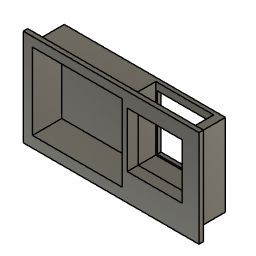
Insert v1 (Autodesk Fusion 360 design; units mm, degrees)
Autodesk Fusion 360 part; units mm, degrees
sketch "Sketch1" plane through (0, 0, 0) normal (0, 1, 0) x (1, 0, 0) in component "Component"
  line L0 (0, 0) -> (240, 0)
  line L1 (240, 0) -> (240, -132)
  line L2 (240, -132) -> (0, -132)
  line L3 (0, -132) -> (0, 0)
  dimension "d1" = 240
  dimension "d2" = 132
  constraint horizontal L0
  constraint vertical L1
  constraint horizontal L2
  constraint vertical L3
  constraint coincident L0.start L3.end
  measures "d1" distance of L0.start L0.end
  measures "d2" distance of L0.start L2.end
extrude "Extrude1" add sketch "Sketch1" along normal blind 6 in component "Component"
sketch "Sketch2" plane through (0, 6, 0) normal (0, 1, 0) x (-1, 0, 0) in component "Component"
  line L0 (0, 132) -> (-240, 132)
  line L1 (-240, 132) -> (-240, 0)
  line L2 (-240, 0) -> (0, 0)
  line L3 (0, 0) -> (0, 132)
  line L4 (-10, 10) -> (-230, 10)
  line L5 (-230, 10) -> (-230, 122)
  line L6 (-230, 122) -> (-10, 122)
  line L7 (-10, 122) -> (-10, 10)
  dimension "d5" = 220
  dimension "d6" = 112
  constraint horizontal L4
  constraint vertical L5
  constraint horizontal L6
  constraint vertical L7
  measures "d5" distance of L4.start L4.end
  measures "d6" distance of L4.start L6.end
extrude "Extrude2" add sketch "Sketch2" along normal blind 40 contours L4 L5 L6 L7 in component "Component"
sketch "Sketch3" plane through (0, 0, 0) normal (0, 1, 0) x (1, 0, 0) in component "Component"
  line L0 (12.5, -119.5) -> (225, -119.5)
  line L1 (225, -119.5) -> (225, -15)
  line L2 (225, -15) -> (12.5, -15)
  line L3 (12.5, -15) -> (12.5, -119.5)
  constraint horizontal L0
  constraint vertical L1
  constraint horizontal L2
  constraint vertical L3
extrude "Extrude3" cut sketch "Sketch3" along normal blind 40 in component "Component"
sketch "Sketch4" plane through (0, 0, 0) normal (0, 1, 0) x (1, 0, 0) in component "Component"
  line L0 (225, -15) -> (185, -15)
  line L1 (185, -15) -> (185, -120)
  line L2 (185, -120) -> (225, -120)
  line L3 (225, -120) -> (225, -15)
  constraint horizontal L0
  constraint vertical L1
  constraint horizontal L2
  constraint vertical L3
extrude "Extrude4" add 1 faces at (225, 13.3333, 84.6667) along direction (-1, 0, 0) blind 90 in component "Component"
sketch "Sketch5" plane through (0, 0, 0) normal (0, 1, 0) x (1, 0, 0) in component "Component"
  line L0 (140, -115) -> (219, -115)
  line L1 (219, -115) -> (219, -35)
  line L2 (219, -35) -> (140, -35)
  line L3 (140, -35) -> (140, -115)
  line L4 (140, -115) -> (220, -115)
  line L5 (220, -115) -> (220, -35)
  line L6 (220, -35) -> (140, -35)
  line L7 (140, -35) -> (140, -115)
  dimension "d13" = 80
  dimension "d14" = 80
  constraint horizontal L0
  constraint vertical L1
  constraint horizontal L2
  constraint vertical L3
  constraint horizontal L4
  constraint vertical L5
  constraint horizontal L6
  constraint vertical L7
  measures "d13" distance of L0.start L4.end
  measures "d14" distance of L0.start L2.end
extrude "Extrude5" cut sketch "Sketch5" along normal blind 50 contours L0 L1 L2 L3 L4 L6 L7 in component "Component"
sketch "Sketch6" plane through (219, 0, 0) normal (-1, 0, 0) x (0, -1, 0) in component "Component"
  line L0 (-46, 115) -> (-46, 35)
  line L1 (-46, 35) -> (0, 35)
  line L2 (0, 35) -> (0, 115)
  line L3 (0, 115) -> (-46, 115)
  line L4 (-46, 35) -> (-41, 35)
  line L5 (-41, 35) -> (-41, 37)
  line L6 (-41, 37) -> (-46, 37)
  line L7 (-46, 37) -> (-46, 35)
  constraint horizontal L4
  constraint vertical L5
  constraint horizontal L6
  constraint vertical L7
  constraint coincident L0.end L1.start
extrude "Extrude6" add sketch "Sketch6" along normal up to surface (79 mm away) contours L0 L1 L4 L5 L6 L7 in component "Component"
sketch "Sketch7" plane through (219, 0, 0) normal (-1, 0, 0) x (0, -1, 0) in component "Component"
  line L0 (-46, 37) -> (-41, 37)
  line L1 (-41, 37) -> (-41, 35)
  line L2 (-41, 35) -> (0, 35)
  line L3 (0, 35) -> (0, 115)
  line L4 (0, 115) -> (-46, 115)
  line L5 (-46, 115) -> (-46, 37)
  line L6 (-41, 37) -> (-15, 37)
  line L7 (-15, 37) -> (-15, 35)
  line L8 (-15, 35) -> (-41, 35)
  line L9 (-41, 35) -> (-41, 37)
  line L10 (-15, 37) -> (0, 37)
  line L11 (0, 37) -> (0, 35)
  line L12 (0, 35) -> (-15, 35)
  line L13 (-15, 35) -> (-15, 37)
  constraint horizontal L6
  constraint vertical L7
  constraint horizontal L8
  constraint vertical L9
  constraint coincident L2 L7.end
  constraint coincident L0.end L1.start
  constraint horizontal L10
  constraint vertical L11
  constraint horizontal L12
  constraint vertical L13
  constraint coincident L2.end L3.start
extrude "Extrude7" add sketch "Sketch7" along normal up to surface (79 mm away) contours L2 L3 L7 L10 L11 L12 L13 in component "Component"
sketch "Sketch8" plane through (0, 0, 37) normal (0, 0, 1) x (-1, 0, 0) in component "Component"
  line L0 (-140, -46) -> (-140, -41)
  line L1 (-140, -41) -> (-219, -41)
  line L2 (-219, -41) -> (-219, -46)
  line L3 (-219, -46) -> (-140, -46)
  line L4 (-215, -39) -> (-212.6, -39)
  line L5 (-212.6, -39) -> (-212.6, -36)
  line L6 (-212.6, -36) -> (-215, -36)
  line L7 (-215, -36) -> (-215, -39)
  line L8 (-215, -36) -> (-217, -36)
  line L9 (-217, -36) -> (-217, -36)
  line L10 (-217, -36) -> (-215, -36)
  line L11 (-215, -36) -> (-215, -36)
  line L12 (-217, -36) -> (-212, -36)
  line L13 (-212, -36) -> (-212, -18)
  line L14 (-212, -18) -> (-217, -18)
  line L15 (-217, -18) -> (-217, -36)
  line L16 (-219, -46) -> (-218, -46)
  line L17 (-218, -46) -> (-218, -41)
  line L18 (-218, -41) -> (-219, -41)
  line L19 (-219, -41) -> (-219, -46)
  constraint horizontal L4
  constraint vertical L5
  constraint horizontal L6
  constraint vertical L7
  constraint horizontal L8
  constraint horizontal L10
  constraint horizontal L12
  constraint vertical L13
  constraint horizontal L14
  constraint vertical L15
  constraint horizontal L16
  constraint vertical L17
  constraint horizontal L18
  constraint vertical L19
  constraint coincident L1 L17.end
  constraint coincident L2.end L3.start
extrude "Extrude8" add sketch "Sketch8" along normal up to surface (78 mm away) contours L1 L2 L3 L16 L17 L18 L19 in component "Component"
sketch "Sketch9" plane through (0, 0, 37) normal (0, 0, 1) x (-1, 0, 0) in component "Component"
  line L0 (-218, -41) -> (-218, -46)
  line L1 (-218, -46) -> (-140, -46)
  line L2 (-140, -46) -> (-140, -41)
  line L3 (-140, -41) -> (-218, -41)
  line L4 (-140, -46) -> (-142, -46)
  line L5 (-142, -46) -> (-142, -41)
  line L6 (-142, -41) -> (-140, -41)
  line L7 (-140, -41) -> (-140, -46)
  line L8 (-218, -41) -> (-219, -41)
  line L9 (-219, -41) -> (-219, -41)
  line L10 (-219, -41) -> (-218, -41)
  line L11 (-218, -41) -> (-218, -41)
  line L12 (-140, -46) -> (-141, -46)
  line L13 (-141, -46) -> (-141, -41)
  line L14 (-141, -41) -> (-140, -41)
  line L15 (-140, -41) -> (-140, -46)
  constraint horizontal L4
  constraint vertical L5
  constraint horizontal L6
  constraint vertical L7
  constraint coincident L3 L5.end
  constraint coincident L1.end L2.start
  constraint horizontal L8
  constraint horizontal L10
  constraint coincident L0.start L3.end
  constraint horizontal L12
  constraint vertical L13
  constraint horizontal L14
  constraint vertical L15
  constraint midpoint L6 L13.end
extrude "Extrude9" add sketch "Sketch9" along normal up to surface (78 mm away) contours L1 L2 L3 L4 L6 L7 L12 L13 L14 L15 in component "Component"
sketch "Sketch10" plane through (0, 0, 115) normal (0, 0, -1) x (1, 0, 0) in component "Component"
  line L0 (141, -41) -> (141, -46)
  line L1 (141, -46) -> (218, -46)
  line L2 (218, -46) -> (218, -41)
  line L3 (218, -41) -> (219, -41)
  line L4 (219, -41) -> (219, 0)
  line L5 (219, 0) -> (140, 0)
  line L6 (140, 0) -> (140, -41)
  line L7 (140, -41) -> (141, -41)
  line L8 (141, -41) -> (218, -41)
  line L9 (218, -41) -> (218, -46)
  line L10 (218, -46) -> (141, -46)
  line L11 (141, -46) -> (141, -41)
  constraint horizontal L8
  constraint vertical L9
  constraint horizontal L10
  constraint vertical L11
  constraint coincident L1.end L2.start
  constraint coincident L0.start L7.end
extrude "Extrude10" add sketch "Sketch10" along normal blind 3 contours L0 L1 L2 L8 L9 L10 L11 in component "Component"
sketch "Sketch11" plane through (0, 0, 37) normal (0, 0, 1) x (-1, 0, 0) in component "Component"
  line L0 (-140, -15) -> (-140, 0)
  line L1 (-140, 0) -> (-219, 0)
  line L2 (-219, 0) -> (-219, -15)
  line L3 (-219, -15) -> (-140, -15)
  line L4 (-140, -15) -> (-141, -15)
  line L5 (-141, -15) -> (-141, 0)
  line L6 (-141, 0) -> (-140, 0)
  line L7 (-140, 0) -> (-140, -15)
  constraint horizontal L4
  constraint vertical L5
  constraint horizontal L6
  constraint vertical L7
  constraint coincident L1 L5.end
  constraint coincident L0.start L3.end
extrude "Extrude11" add sketch "Sketch11" along normal up to surface (78 mm away) contours L0 L1 L3 L4 L5 L6 L7 in component "Component"
sketch "Sketch12" plane through (0, 0, 37) normal (0, 0, 1) x (-1, 0, 0) in component "Component"
  line L0 (-141, -15) -> (-141, 0)
  line L1 (-141, 0) -> (-219, 0)
  line L2 (-219, 0) -> (-219, -15)
  line L3 (-219, -15) -> (-141, -15)
  line L4 (-219, -15) -> (-218, -15)
  line L5 (-218, -15) -> (-218, 0)
  line L6 (-218, 0) -> (-219, 0)
  line L7 (-219, 0) -> (-219, -15)
  constraint horizontal L4
  constraint vertical L5
  constraint horizontal L6
  constraint vertical L7
  constraint coincident L1 L5.end
  constraint coincident L2.end L3.start
extrude "Extrude12" add sketch "Sketch12" along normal up to surface (78 mm away) contours L1 L2 L3 L4 L5 L6 L7 in component "Component"
sketch "Sketch13" plane through (0, 0, 115) normal (0, 0, -1) x (1, 0, 0) in component "Component"
  line L0 (218, -15) -> (218, 0)
  line L1 (218, 0) -> (141, 0)
  line L2 (141, 0) -> (141, -15)
  line L3 (141, -15) -> (140, -15)
  line L4 (140, -15) -> (140, -41)
  line L5 (140, -41) -> (219, -41)
  line L6 (219, -41) -> (219, -15)
  line L7 (219, -15) -> (218, -15)
  line L8 (164, 63) -> (166, 63)
  line L9 (166, 63) -> (166, 78)
  line L10 (166, 78) -> (164, 78)
  line L11 (164, 78) -> (164, 63)
  line L12 (141, 0) -> (218, 0)
  line L13 (218, 0) -> (218, -15)
  line L14 (218, -15) -> (141, -15)
  line L15 (141, -15) -> (141, 0)
  constraint horizontal L8
  constraint vertical L9
  constraint horizontal L10
  constraint vertical L11
  constraint horizontal L12
  constraint vertical L13
  constraint horizontal L14
  constraint vertical L15
  constraint coincident L0.start L7.end
  constraint coincident L1.end L2.start
extrude "Extrude13" add sketch "Sketch13" along normal blind 3 contours L0 L1 L2 L12 L13 L14 L15 in component "Component"
extrude "Extrude14" cut 1 faces at (192.3333, 23.6667, 115) along direction (0, 0, 1) blind 43 in component "Component"
extrude "Extrude15" add 1 faces at (218, 10, 87) along direction (-1, 0, 0) blind 1 in component "Component"
extrude "Extrude16" add 1 faces at (218, 44.3333, 62) along direction (-1, 0, 0) blind 1 in component "Component"
extrude "Extrude17" add 1 faces at (141, 10, 87) along direction (1, 0, 0) blind 1 in component "Component"
extrude "Extrude18" add 1 faces at (141, 44.3333, 87) along direction (1, 0, 0) blind 1 in component "Component"
component "Insert" placed x (1, 0, 0) y (0, 1, 0) z (0, 0, 1) at (0, 0, 0)
component "Component" placed x (1, 0, 0) y (0, 1, 0) z (0, 0, 1) at (0, 0, 0) in component "Insert"
